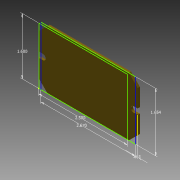
# Autodesk Inventor part: ElectronicsBoard
Saved by Autodesk Inventor 2012 (Build 160160000, 160)
## iProperties
Created: 2012-04-11
Part Number: ElectronicsBoard
Material: Phenolic
Document SubType Name: Modeling
Designer: Admin
Mass: 6.27604 g
Surface Area: 60.9103 cm^2
Volume: 4.54785 cm^3
Density: 1.38 g/cm^3
Author: Admin
Autodesk Inventor part; units mm, degrees
ref_plane "YZ Plane" through (0, 0, 0) normal (1, 0, 0) x (0, 1, 0)
ref_plane "XZ Plane" through (0, 0, 0) normal (0, 1, 0) x (-1, 0, 0)
ref_plane "XY Plane" through (0, 0, 0) normal (0, 0, 1) x (1, 0, 0)
sketch "Sketch1" plane through (0, 0, 0) normal (0, 0, 1) x (1, 0, 0)
  line L0 (0, 0) -> (71, 0)
  line L1 (71, 0) -> (71, 42)
  line L2 (71, 42) -> (0, 42)
  line L3 (0, 42) -> (0, 0)
  dimension "d0" = 71
  dimension "d1" = 42
  constraints: 8 end point, 2 parallel, 1 horizontal, 1 perpendicular
  measures "d0" distance of L2.end L1.end
  measures "d1" distance between parallel lines of L2 L0
extrude "Extrusion1" add sketch "Sketch1" along normal blind 1.5875
chamfer "Chamfer1" distance 6.35 angle 45 4 edges at (0, 42, 0.7937) (0, 0, 0.7937) (71, 0, 0.7937) (71, 42, 0.7937)
sketch "Sketch2" plane through (0, 0, 1.5875) normal (0, 0, 1) x (1, 0, 0)
  line L0 (0, 6.35) -> (0, 35.65) projected
  line L1 (71, 35.65) -> (71, 6.35) projected
  circle A0 centre (3, 21) radius 2
  circle A1 centre (68, 21) radius 2
  line L2 (5, 21) -> (5, 26.1458)
  line L3 (3, 23) -> (0, 23)
  line L4 (3, 19) -> (0, 19)
  line L5 (66, 18.2827) -> (66, 24.0716)
  line L6 (68, 23) -> (71, 23)
  line L7 (68, 19) -> (71, 19)
  line L8 (71, 19) -> (71, 23)
  line L9 (0, 19) -> (0, 23)
  point P0 (0, 0)
  dimension "d7" = 4
  dimension "d8" = 4
  dimension "d10" = 5
  dimension "d11" = 5
  constraints: 16 end point, 6 tangent, 5 point on circle, 4 perpendicular, 4 point on line, 2 centre point, 2 collinear, 2 parallel
  measures "d7" diameter of A0
  measures "d8" diameter of A1
  measures "d10" distance between parallel lines of L0 L2
  measures "d11" distance between parallel lines of L1 L5
extrude "Extrusion2" cut sketch "Sketch2" against normal blind 1.5875
sketch "Sketch3" plane through (0, 0, 1.5875) normal (0, 0, 1) x (1, 0, 0)
  line L0 (71, 19) -> (71, 6.35) projected
  line L1 (1.5875, 42) -> (69.4125, 42)
  line L2 (69.4125, 42) -> (69.4125, 0)
  line L3 (69.4125, 0) -> (1.5875, 0)
  line L4 (1.5875, 0) -> (1.5875, 42)
  line L5 (0, 40.64) -> (63.5, 40.64)
  line L6 (63.5, 40.64) -> (63.5, 0)
  line L7 (63.5, 0) -> (0, 0)
  line L8 (0, 0) -> (0, 40.64)
  point P0 (0, 0)
  dimension "d14" = 67.825
  dimension "d15" = 1.5875
  dimension "d16" = 63.5
  dimension "d17" = 42
  dimension "d18" = 40.64
  constraints: 16 end point, 4 parallel, 2 horizontal, 2 perpendicular
  measures "d14" distance between parallel lines of L2 L4
  measures "d15" distance between parallel lines of L0 L2
  measures "d16" distance between parallel lines of L6 L8
  measures "d17" distance between parallel lines of L1 L3
  measures "d18" distance between parallel lines of L7 L5
body "Solid1"
